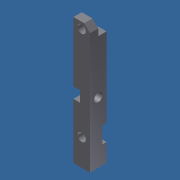
# Autodesk Inventor part: CHASSI ESQUERDO(37)
Saved by Autodesk Inventor 2012 SP1 (Build 160190100, 190)
## iProperties
Created: 2012-07-23
Part Number: CHASSI ESQUERDO(37)
Material: Carbon Steel
Document SubType Name: Modeling
Designer: bruno.silveira
Mass: 480.07 g
Surface Area: 130 cm^2
Volume: 61 cm^3
Density: 7.87 g/cm^3
Author: bruno.silveira
Autodesk Inventor part; units mm, degrees
ref_plane "YZ Plane" through (0, 0, 0) normal (1, 0, 0) x (0, 1, 0)
ref_plane "XZ Plane" through (0, 0, 0) normal (0, 1, 0) x (-1, 0, 0)
ref_plane "XY Plane" through (0, 0, 0) normal (0, 0, 1) x (1, 0, 0)
sketch "Sketch1" plane through (0, 0, 0) normal (0, 0, 1) x (1, 0, 0)
  line L0 (0, 0) -> (20, 0)
  line L1 (20, 0) -> (20, 20)
  line L2 (20, 20) -> (0, 20)
  line L3 (0, 20) -> (0, 0)
  dimension "d0" = 20
  dimension "d1" = 20
  constraints: 8 end point, 2 parallel, 1 horizontal, 1 perpendicular
  measures "d0" distance of L0.end L1.end
  measures "d1" distance of L1.end L2.end
extrude "Extrusion1" add sketch "Sketch1" along normal blind 152.5
sketch "Sketch2" plane through (0, 20, 0) normal (0, 1, 0) x (1, 0, 0)
  line L0 (0, -152.5) -> (20, -152.5) projected
  line L1 (0, 0) -> (0, -152.5) projected
  line L2 (0, -80) -> (8, -80)
  line L3 (8, -80) -> (8, -67)
  line L4 (8, -67) -> (0, -67)
  line L5 (0, -67) -> (0, -80)
  dimension "d4" = 13
  dimension "d5" = 72.5
  dimension "d6" = 8
  constraints: 8 end point, 2 parallel, 1 horizontal, 1 perpendicular, 1 point on line
  measures "d4" distance of L4.end L2.start
  measures "d5" distance between parallel lines of L0 L2
  measures "d6" distance between parallel lines of L1 L3
extrude "Extrusion2" cut sketch "Sketch2" against normal blind 20
sketch "Sketch3" plane through (0, 20, 0) normal (0, 1, 0) x (1, 0, 0)
  line L0 (0, -80) -> (0, -152.5) projected
  line L1 (0, -152.5) -> (20, -152.5) projected
  line L2 (20, 0) -> (20, -152.5) projected
  line L3 (0, -137.5) -> (20, -137.5)
  dimension "d9" = 15
  constraints: 2 end point, 2 point on line, 1 perpendicular
  measures "d9" distance between parallel lines of L1 L3
extrude "Extrusion3" cut sketch "Sketch3" against normal blind 10
chamfer "Chamfer1" distance 7 angle 45 1 edges at (20, 5, 152.5)
sketch "Sketch4" plane through (0, 20, 0) normal (0, 1, 0) x (1, 0, 0)
  line L0 (0, -137.5) -> (10, -137.5)
  line L1 (10, -137.5) -> (10, -112.5)
  line L2 (10, -112.5) -> (0, -112.5)
  line L3 (0, -112.5) -> (0, -137.5)
  dimension "d15" = 10
  dimension "d16" = 25
  constraints: 8 end point, 2 parallel, 1 horizontal, 1 perpendicular
  measures "d15" distance of L0.start L0.end
  measures "d16" distance of L0.end L1.end
extrude "Extrusion4" cut sketch "Sketch4" against normal blind 10
chamfer "Chamfer2" distance 10 angle 45 1 edges at (10, 10, 125)
sketch "Sketch5" plane through (0, 0, 0) normal (0, -1, 0) x (1, 0, 0)
  line L0 (0, 80) -> (0, 152.5) projected
  line L1 (20, 137.5) -> (0, 137.5) projected
  point P0 (10, 145)
  dimension "d22" = 10
  dimension "d23" = 7.5
  measures "d22" distance from line of L0 point (10, 145)
  measures "d23" distance from line of L1 point (10, 145)
hole "Hole1" at (10, 0, 145) direction (0, 1, 0) diameter 6.5 depth 10 tip angle 118 counterbore diameter 10 counterbore depth 7
sketch "Sketch6" plane through (20, 0, 0) normal (1, 0, 0) x (0, 0, -1)
  line L0 (0, 0) -> (-145.5, 0) projected
  line L1 (-80, 20) -> (-80, 0) projected
  line L2 (-67, 20) -> (-67, 0) projected
  line L3 (-152.5, 10) -> (-152.5, 0) projected
  point P0 (-73.5, 10)
  dimension "d31" = 79
  dimension "d32" = 10
  measures "d31" distance from line of L3 point (-73.5, 10)
  measures "d32" distance from line of L0 point (-73.5, 10)
hole "Hole2" at (20, 10, 73.5) direction (-1, 0, 0) diameter 6.5 depth 13 tip angle 118 counterbore diameter 10 counterbore depth 7
sketch "Sketch7" plane through (0, 0, 0) normal (-1, 0, 0) x (0, 0, 1)
  line L0 (0, 20) -> (67, 20) projected
  line L1 (0, 20) -> (0, 0) projected
  line L2 (42, 20) -> (22, 20)
  line L3 (22, 20) -> (22, 15)
  line L4 (22, 15) -> (42, 15)
  line L5 (42, 15) -> (42, 20)
  dimension "d40" = 20
  dimension "d41" = 22
  dimension "d42" = 5
  constraints: 8 end point, 2 parallel, 1 horizontal, 1 perpendicular, 1 point on line
  measures "d40" distance of L3.end L4.end
  measures "d41" distance between parallel lines of L1 L3
  measures "d42" distance between parallel lines of L0 L4
extrude "Extrusion5" cut sketch "Sketch7" against normal blind 20
sketch "Sketch8" plane through (0, 0, 0) normal (0, -1, 0) x (1, 0, 0)
  line L0 (20, 0) -> (20, 145.5) projected
  line L1 (0, 22) -> (20, 22) projected
  line L2 (0, 42) -> (20, 42) projected
  point P0 (10, 32)
  dimension "d45" = 10
  dimension "d46" = 10
  measures "d45" distance from line of L0 point (10, 32)
  measures "d46" distance from line of L2 point (10, 32)
hole "Hole3" at (10, 0, 32) direction (0, 1, 0) diameter 6.5 depth 15 tip angle 118 counterbore diameter 10 counterbore depth 7
sketch "Sketch9" plane through (0, 0, 0) normal (-1, 0, 0) x (0, 0, 1)
  line L0 (0, 0) -> (67, 0) projected
  line L1 (42, 15) -> (22, 15) projected
  line L2 (27, 7) -> (27, 0) projected
  line L3 (27, 7) -> (37, 7) projected
  line L4 (37, 7) -> (37, 0) projected
  line L5 (35.25, 15) -> (35.25, 7) projected
  line L6 (28.75, 15) -> (28.75, 7) projected
  line L7 (32, 15) -> (32, 0)
  point P0 (39.5, 10)
  point P1 (24.5, 10)
  dimension "d54" = 15
  dimension "d56" = 7.5
  dimension "d57" = 10
  constraints: 2 end point, 1 midpoint
  measures "d54" distance of point (39.5, 10) point (24.5, 10)
  measures "d56" horizontal distance of L7.end point (24.5, 10)
  measures "d57" distance from line of L0 point (24.5, 10)
hole "Hole4" at (0, 10, 39.5) at (0, 10, 24.5) direction (1, 0, 0) diameter 3.2 depth 12 tip angle 118
sketch "Sketch10" plane through (0, 0, 0) normal (0, 0, -1) x (-1, 0, 0)
  line L0 (-20, 20) -> (0, 20) projected
  line L1 (-20, 0) -> (-20, 20) projected
  point P0 (-13, 10)
  dimension "d65" = 7
  dimension "d66" = 10
  measures "d65" distance from line of L1 point (-13, 10)
  measures "d66" distance from line of L0 point (-13, 10)
hole "Hole5" at (13, 10, 0) direction (0, 0, 1) diameter 4.917 depth 8 tip angle 118 thread size "M6x1" class "6H" standard "ANSI Metric M Profile"
chamfer "Chamfer3" distance 0.5 angle 45 1 edges at (13, 7.5415, 0)
sketch "Sketch11" plane through (0, 0, 0) normal (-1, 0, 0) x (0, 0, 1)
  line L0 (0, 20) -> (22, 20) projected
  line L1 (0, 20) -> (0, 0) projected
  point P0 (6.5, 10)
  dimension "d77" = 10
  dimension "d78" = 6.5
  measures "d77" distance from line of L0 point (6.5, 10)
  measures "d78" distance from line of L1 point (6.5, 10)
hole "Hole6" at (0, 10, 6.5) direction (1, 0, 0) diameter 4.917 depth 8 tip angle 118 thread size "M6x1" class "6H" standard "ANSI Metric M Profile"
chamfer "Chamfer4" distance 0.5 angle 45 1 edges at (0, 10, 4.0415)
body "Solid1"
